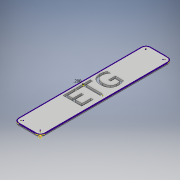
# Autodesk Inventor part: EtgSignModV3
Saved by Autodesk Inventor 2019 (Build 230136000, 136)
## iProperties
Created: 2018-10-30
Part Number: EtgSignModV3
Material: Generic
Document SubType Name: Modeling
Designer: Administrator
Density: 1 g/cm^3
Appearance: Default
Author: Administrator
Autodesk Inventor part; units mm, degrees
ref_plane "YZ Plane" through (0, 0, 0) normal (1, 0, 0) x (0, 1, 0)
ref_plane "XZ Plane" through (0, 0, 0) normal (0, 1, 0) x (-1, 0, 0)
ref_plane "XY Plane" through (0, 0, 0) normal (0, 0, 1) x (1, 0, 0)
sketch "Sketch1" plane through (0, 0, 0) normal (0, 1, 0) x (-1, 0, 0)
  line L0 (53.975, 0) -> (250.825, 0)
  line L1 (304.8, -53.975) -> (304.8, -1470.025)
  line L2 (250.825, -1524) -> (53.975, -1524)
  line L3 (0, -1470.025) -> (0, -53.975)
  circle A0 centre (263.525, -41.275) radius 5.5563
  circle A1 centre (263.525, -762) radius 5.5563
  circle A2 centre (263.525, -1482.725) radius 5.5563
  circle A3 centre (41.275, -41.275) radius 5.5563
  circle A4 centre (41.275, -762) radius 5.5563
  circle A5 centre (41.275, -1482.725) radius 5.5563
  arc A6 (304.8, -53.975) -> (250.825, 0) centre (250.825, -53.975) ccw
  arc A7 (0, -1470.025) -> (53.975, -1524) centre (53.975, -1470.025) ccw
  arc A8 (250.825, -1524) -> (304.8, -1470.025) centre (250.825, -1470.025) ccw
  arc A9 (53.975, 0) -> (0, -53.975) centre (53.975, -53.975) ccw
  point P0 (0, 0)
  point P1 (304.8, -1524)
  point P2 (0, -1524)
  dimension "d0" = 304.8
  dimension "d1" = 1524
  dimension "d2" = 11.1125
  dimension "d5" = 720.725
  dimension "d8" = 222.25
  dimension "d11" = 41.275
  dimension "d12" = 41.275
  dimension "d13" = 53.975
  constraints: 10 centre point, 8 end point, 8 point on circle, 8 tangent, 6 point on line, 3 equal radius, 2 horizontal, 2 parallel, 1 perpendicular, 1 vertical, 10 other
  measures "d0" distance of point (304.8, -1524) point (0, -1524)
  measures "d1" distance between parallel lines of L2 L0
  measures "d2" diameter of A0
  measures "d5" distance of A0.centre A1.centre
  measures "d8" distance of A0.centre A3.centre
  measures "d11" distance from line of L0 A0.centre
  measures "d12" distance from line of L1 A0.centre
  measures "d13" radius of A6
extrude "Extrusion1" add sketch "Sketch1" along normal blind 22.225
ref_plane "Work Plane3" through (0, 17.4625, 0) normal (0, 1, 0) x (1, 0, 0)
sketch "Sketch2" plane through (0, 17.4625, 0) normal (0, 1, 0) x (1, 0, 0)
  circle A0 centre (-41.275, 1482.725) radius 5.5562 projected
  circle A1 centre (-41.275, 762) radius 5.5562 projected
  circle A2 centre (-41.275, 41.275) radius 5.5562 projected
  circle A3 centre (-263.525, 1482.725) radius 5.5562 projected
  circle A4 centre (-263.525, 762) radius 5.5562 projected
  circle A5 centre (-263.525, 41.275) radius 5.5562 projected
  line L0 (-250.825, 0) -> (-53.975, 0) projected
  arc A6 (-53.975, 0) -> (0, 53.975) centre (-53.975, 53.975) ccw projected
  line L1 (0, 53.975) -> (0, 1470.025) projected
  arc A7 (0, 1470.025) -> (-53.975, 1524) centre (-53.975, 1470.025) ccw projected
  line L2 (-53.975, 1524) -> (-250.825, 1524) projected
  arc A8 (-250.825, 1524) -> (-304.8, 1470.025) centre (-250.825, 1470.025) ccw projected
  line L3 (-304.8, 1470.025) -> (-304.8, 53.975) projected
  arc A9 (-304.8, 53.975) -> (-250.825, 0) centre (-250.825, 53.975) ccw projected
  line L4 (0, 53.975) -> (0, 1470.025)
  arc A10 (-250.825, 1524) -> (-304.8, 1470.025) centre (-250.825, 1470.025) ccw projected
  line L5 (-53.975, 1524) -> (-250.825, 1524)
  line L6 (-304.8, 1470.025) -> (-304.8, 53.975) projected
  line L7 (-304.8, 1470.025) -> (-304.8, 53.975)
  line L8 (-250.825, 0) -> (-53.975, 0)
  point P0 (0, 0)
  constraints: 8 end point, 2 horizontal, 2 vertical, 1 tangent
ref_plane "Work Plane4" through (0, 4.7625, 0) normal (0, -1, 0) x (1, 0, 0)
sketch "Sketch3" plane through (0, 4.7625, 0) normal (0, -1, 0) x (1, 0, 0)
  circle A0 centre (-41.275, -1482.725) radius 5.5562 projected
  circle A1 centre (-41.275, -762) radius 5.5562 projected
  circle A2 centre (-41.275, -41.275) radius 5.5562 projected
  circle A3 centre (-263.525, -1482.725) radius 5.5562 projected
  circle A4 centre (-263.525, -762) radius 5.5562 projected
  circle A5 centre (-263.525, -41.275) radius 5.5562 projected
  line L0 (-250.825, 0) -> (-53.975, 0) projected
  arc A6 (0, -53.975) -> (-53.975, 0) centre (-53.975, -53.975) ccw projected
  line L1 (0, -53.975) -> (0, -1470.025) projected
  arc A7 (-53.975, -1524) -> (0, -1470.025) centre (-53.975, -1470.025) ccw projected
  line L2 (-53.975, -1524) -> (-250.825, -1524) projected
  arc A8 (-304.8, -1470.025) -> (-250.825, -1524) centre (-250.825, -1470.025) ccw projected
  line L3 (-304.8, -1470.025) -> (-304.8, -53.975) projected
  arc A9 (-250.825, 0) -> (-304.8, -53.975) centre (-250.825, -53.975) ccw projected
  line L4 (-299.72, -53.975) -> (-299.72, -1470.025)
  arc A10 (-299.72, -1470.025) -> (-250.825, -1518.92) centre (-250.825, -1470.025) ccw
  line L5 (-250.825, -1518.92) -> (-53.975, -1518.92)
  arc A11 (-53.975, -1518.92) -> (-5.08, -1470.025) centre (-53.975, -1470.025) ccw
  line L6 (-5.08, -1470.025) -> (-5.08, -53.975)
  arc A12 (-5.08, -53.975) -> (-53.975, -5.08) centre (-53.975, -53.975) ccw
  line L7 (-53.975, -5.08) -> (-250.825, -5.08)
  arc A13 (-250.825, -5.08) -> (-299.72, -53.975) centre (-250.825, -53.975) ccw
  point P0 (0, 0)
  dimension "d26" = 5.08
  constraints: 8 end point, 8 point on circle, 4 centre point, 7 other
  measures "d26" distance between parallel lines of L3 L4
sketch "Sketch8" plane through (0, 22.225, 0) normal (0, 1, 0) x (1, 0, 0)
  arc A0 (-53.975, 0) -> (0, 53.975) centre (-53.975, 53.975) ccw projected
  line L0 (-250.825, 0) -> (-53.975, 0) projected
  line L1 (-53.975, 0) -> (-250.825, 0)
  arc A1 (-304.8, 53.975) -> (-250.825, 0) centre (-250.825, 53.975) ccw projected
  arc A2 (-250.825, 1524) -> (-304.8, 1470.025) centre (-250.825, 1470.025) ccw projected
  line L2 (-304.8, 53.975) -> (-304.8, 1470.025)
  line L3 (-53.975, 1524) -> (-250.825, 1524) projected
  line L4 (-250.825, 1524) -> (-53.975, 1524)
  arc A3 (0, 1470.025) -> (-53.975, 1524) centre (-53.975, 1470.025) ccw projected
  line L5 (0, 1470.025) -> (0, 53.975)
  arc A4 (-53.975, 0) -> (0, 53.975) centre (-53.975, 53.975) ccw
  arc A5 (-304.8, 53.975) -> (-250.825, 0) centre (-250.825, 53.975) ccw
  arc A6 (-250.825, 1524) -> (-304.8, 1470.025) centre (-250.825, 1470.025) ccw
  arc A7 (0, 1470.025) -> (-53.975, 1524) centre (-53.975, 1470.025) ccw
  line L6 (-299.72, 1470.025) -> (-299.72, 53.975)
  arc A8 (-299.72, 53.975) -> (-250.825, 5.08) centre (-250.825, 53.975) ccw
  line L7 (-250.825, 5.08) -> (-53.975, 5.08)
  arc A9 (-53.975, 5.08) -> (-5.08, 53.975) centre (-53.975, 53.975) ccw
  line L8 (-5.08, 53.975) -> (-5.08, 1470.025)
  arc A10 (-5.08, 1470.025) -> (-53.975, 1518.92) centre (-53.975, 1470.025) ccw
  line L9 (-53.975, 1518.92) -> (-250.825, 1518.92)
  arc A11 (-250.825, 1518.92) -> (-299.72, 1470.025) centre (-250.825, 1470.025) ccw
  point P0 (0, 0)
  dimension "d25" = 5.08
  constraints: 16 end point, 16 point on circle, 9 tangent, 8 centre point, 2 horizontal, 2 vertical, 7 other
  measures "d25" distance between parallel lines of L2 L6
extrude "Extrusion2" cut sketch "Sketch3" against normal blind 12.7 contours L0 A6 L1 A7 L2 A8 L3 A9
sketch "Sketch9" plane through (0, 22.225, 0) normal (0, 1, 0) x (1, 0, 0)
  line L0 (-218.0203, 368.0695) -> (-210.4225, 368.0695) construction
  line L1 (-210.4225, 368.0695) -> (-210.4225, 364.9079) construction
  line L2 (-210.4225, 364.9079) -> (-218.0203, 364.9079) construction
  line L3 (-218.0203, 364.9079) -> (-218.0203, 368.0695) construction
  line L4 (173.3464, 113.7892) -> (180.9442, 113.7892) construction
  line L5 (180.9442, 113.7892) -> (180.9442, 110.6276) construction
  line L6 (180.9442, 110.6276) -> (173.3464, 110.6276) construction
  line L7 (173.3464, 110.6276) -> (173.3464, 113.7892) construction
  line L8 (-274.32, 513.08) -> (-274.32, 13174.4282) construction
  line L9 (-274.32, 13174.4282) -> (8922.6527, 13174.4282) construction
  line L10 (8922.6527, 13174.4282) -> (8922.6527, 513.08) construction
  line L11 (8922.6527, 513.08) -> (-274.32, 513.08) construction
  line L12 (-251.3686, 562.4549) -> (-240.4288, 562.4549) construction
  line L13 (-240.4288, 562.4549) -> (-240.4288, 562.4549) construction
  line L14 (-240.4288, 562.4549) -> (-251.3686, 562.4549) construction
  line L15 (-251.3686, 562.4549) -> (-251.3686, 562.4549) construction
  line L16 (-299.72, 53.975) -> (-299.72, 1470.025) projected
  line L17 (-250.825, 0) -> (-53.975, 0) projected
  line L18 (-57.1562, 534.6926) -> (-270.5162, 534.6926)
  line L19 (-270.5162, 534.6926) -> (-270.5162, 668.1723)
  line L20 (-270.5162, 668.1723) -> (-245.2726, 668.1723)
  line L21 (-245.2726, 668.1723) -> (-245.2726, 563.0484)
  line L22 (-245.2726, 563.0484) -> (-186.832, 563.0484)
  line L23 (-186.832, 563.0484) -> (-186.832, 661.0834)
  line L24 (-186.832, 661.0834) -> (-161.5885, 661.0834)
  line L25 (-161.5885, 661.0834) -> (-161.5885, 563.0484)
  line L26 (-161.5885, 563.0484) -> (-82.3997, 563.0484)
  line L27 (-82.3997, 563.0484) -> (-82.3997, 668.1723)
  line L28 (-82.3997, 668.1723) -> (-57.1562, 668.1723)
  line L29 (-57.1562, 668.1723) -> (-57.1562, 534.6926)
  line L30 (-57.1562, 749.0901) -> (-245.2726, 749.0901)
  line L31 (-245.2726, 749.0901) -> (-245.2726, 677.509)
  line L32 (-245.2726, 677.509) -> (-270.5162, 677.509)
  line L33 (-270.5162, 677.509) -> (-270.5162, 849.0269)
  line L34 (-270.5162, 849.0269) -> (-245.2726, 849.0269)
  line L35 (-245.2726, 849.0269) -> (-245.2726, 777.4458)
  line L36 (-245.2726, 777.4458) -> (-57.1562, 777.4458)
  line L37 (-57.1562, 777.4458) -> (-57.1562, 749.0901)
  spline S0 degree 2 poles (-53.0065, 960.0294) (-53.0065, 937.3794) (-66.8386, 899.8598) (-80.8436, 886.3736) knots 0 0 0 1 2 2 2
  spline S1 degree 2 poles (-80.8436, 886.3736) (-95.0215, 872.8873) (-136.8636, 858.5365) (-164.0091, 858.5365) knots 0 0 0 1 2 2 2
  spline S2 degree 2 poles (-164.0091, 858.5365) (-189.7713, 858.5365) (-230.576, 873.0602) (-245.0997, 886.5465) knots 0 0 0 1 2 2 2
  spline S3 degree 2 poles (-245.0997, 886.5465) (-259.1047, 899.514) (-274.32, 937.5523) (-274.32, 960.2023) knots 0 0 0 1 2 2 2
  spline S4 degree 2 poles (-274.32, 960.2023) (-274.32, 971.0951) (-271.2078, 990.8058) (-268.4414, 999.7967) knots 0 0 0 1 2 2 2
  spline S5 degree 2 poles (-268.4414, 999.7967) (-266.3665, 1007.0586) (-258.7589, 1024.6945) (-255.9925, 1030.0544) knots 0 0 0 1 2 2 2
  line L38 (-255.9925, 1030.0544) -> (-221.7581, 1030.0544)
  line L39 (-221.7581, 1030.0544) -> (-221.7581, 1027.6338)
  spline S6 degree 2 poles (-221.7581, 1027.6338) (-226.4264, 1022.2739) (-234.8985, 1011.0353) (-239.7398, 1000.6612) knots 0 0 0 1 2 2 2
  spline S7 degree 2 poles (-239.7398, 1000.6612) (-244.0623, 992.0162) (-249.768, 969.7119) (-249.768, 956.9172) knots 0 0 0 1 2 2 2
  spline S8 degree 2 poles (-249.768, 956.9172) (-249.768, 926.1408) (-203.4305, 888.1026) (-164.8736, 888.1026) knots 0 0 0 1 2 2 2
  spline S9 degree 2 poles (-164.8736, 888.1026) (-143.4338, 888.1026) (-111.2742, 898.1308) (-100.2086, 907.6404) knots 0 0 0 1 2 2 2
  spline S10 degree 2 poles (-100.2086, 907.6404) (-89.1429, 916.8042) (-77.5585, 942.7393) (-77.5585, 958.992) knots 0 0 0 1 2 2 2
  spline S11 degree 2 poles (-77.5585, 958.992) (-77.5585, 970.9222) (-81.0165, 994.7826) (-84.4746, 1002.9089) knots 0 0 0 1 2 2 2
  line L40 (-84.4746, 1002.9089) -> (-139.63, 1002.9089)
  line L41 (-139.63, 1002.9089) -> (-139.63, 953.4592)
  line L42 (-139.63, 953.4592) -> (-164.5278, 953.4592)
  line L43 (-164.5278, 953.4592) -> (-164.5278, 1030.9189)
  line L44 (-164.5278, 1030.9189) -> (-71.3341, 1030.9189)
  spline S12 degree 2 poles (-71.3341, 1030.9189) (-68.9134, 1025.559) (-61.4787, 1007.2315) (-59.231, 999.4509) knots 0 0 0 1 2 2 2
  spline S13 degree 2 poles (-59.231, 999.4509) (-56.1188, 988.9039) (-53.0065, 971.9596) (-53.0065, 960.0294) knots 0 0 0 1 2 2 2
  point P0 (0, 0)
  dimension "d29" = 25.4
  dimension "d30" = 513.08
  constraints: 8 other
  measures "d29" distance between parallel lines of L16 L8
  measures "d30" distance between parallel lines of L17 L11
extrude "Extrusion3" cut sketch "Sketch9" against normal blind 25.4
body "Solid1"
